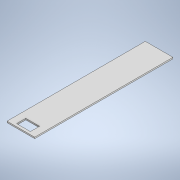
# Autodesk Inventor part: Pieza2
Saved by Autodesk Inventor 2020.5 (Build 245400000, 400)
## iProperties
Created: 2023-01-30
Part Number: Pieza2
Material: Genérico
Document SubType Name: Modeling
Designer: André Aguirre Apolo
Density: 1 g/cm^3
Appearance: Valor por defecto
Author: André Aguirre Apolo
Autodesk Inventor part; units mm, degrees
ref_plane "YZ Plane" through (0, 0, 0) normal (1, 0, 0) x (0, 1, 0)
ref_plane "XZ Plane" through (0, 0, 0) normal (0, 1, 0) x (-1, 0, 0)
ref_plane "XY Plane" through (0, 0, 0) normal (0, 0, 1) x (1, 0, 0)
sketch "Boceto1" plane through (0, 0, 0) normal (0, 1, 0) x (-1, 0, 0)
  point P0 (0, 0)
sketch "Boceto2" plane through (0, 0, 0) normal (0, 1, 0) x (-1, 0, 0)
  line L0 (-76.2, 381) -> (76.2, 381)
  line L1 (76.2, 381) -> (76.2, -381)
  line L2 (76.2, -381) -> (-76.2, -381)
  line L3 (-76.2, -381) -> (-76.2, 381)
  line L4 (-76.2, 381) -> (76.2, -381) construction
  line L5 (76.2, 381) -> (-76.2, -381) construction
  point P0 (0, 0)
  dimension "d0" = 152.4
  dimension "d1" = 762
  constraints: 12 end point, 2 midpoint, 2 parallel, 1 horizontal, 1 perpendicular
  measures "d0" distance of L1.end L2.end
  measures "d1" distance of L0.end L1.end
extrude "Extrusión1" add sketch "Boceto2" along normal mid plane 7.62
sketch "Boceto3" plane through (0, 3.81, 0) normal (0, 1, 0) x (1, 0, 0)
  line L0 (-76.2, -381) -> (76.2, -381) projected
  line L1 (38.1, -315.722) -> (-38.1, -315.722)
  line L2 (-38.1, -315.722) -> (-38.1, -366.522)
  line L3 (-38.1, -366.522) -> (38.1, -366.522)
  line L4 (38.1, -366.522) -> (38.1, -315.722)
  line L5 (38.1, -315.722) -> (-38.1, -366.522) construction
  line L6 (-38.1, -315.722) -> (38.1, -366.522) construction
  point P0 (0, 0)
  point P1 (0, -366.522)
  point P2 (0, -341.122)
  dimension "d4" = 14.478
  dimension "d5" = 76.2
  dimension "d6" = 50.8
  dimension "d7" = 0
  constraints: 12 end point, 2 midpoint, 2 parallel, 1 horizontal, 1 perpendicular
  measures "d4" distance from line of L0 point (0, -366.522)
  measures "d5" distance of L3.end L2.end
  measures "d6" distance of L2.end L1.end
  measures "d7" distance from line of point (0, -366.522) L3
extrude "Extrusión2" cut sketch "Boceto3" against normal blind 25.4
